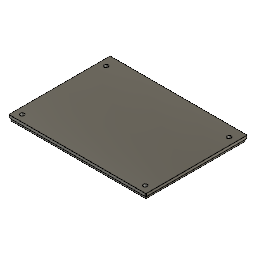
Final Board and Enclosure v2 (Autodesk Fusion 360 archive; units mm, degrees)
design "Lid"
Autodesk Fusion 360 part; units mm, degrees
sketch "Sketch 2" plane through (0, 0, 0) normal (0, 0, 1) x (1, 0, 0)
  circle A0 centre (5, 80) radius 1.75
  line L0 (-0.1, -0.1) -> (120.73, -0.1)
  arc A1 (-0.6, -1.1) -> (-1.1, -0.6) centre (-0.6, -0.6) cw
  line L1 (-1.1, -0.6) -> (-1.1, 89.17)
  arc A2 (-1.1, 89.17) -> (-0.6, 89.67) centre (-0.6, 89.17) cw
  line L2 (121.73, 89.17) -> (121.73, -0.6)
  circle A3 centre (115, 80) radius 1.75
  line L3 (120.73, -0.1) -> (120.73, 88.67)
  line L4 (120.73, 88.67) -> (-0.1, 88.67)
  circle A4 centre (115, 5) radius 1.75
  circle A5 centre (5, 5) radius 1.75
  line L5 (121.23, -1.1) -> (-0.6, -1.1)
  arc A6 (121.23, 89.67) -> (121.73, 89.17) centre (121.23, 89.17) cw
  line L6 (-0.1, 88.67) -> (-0.1, -0.1)
  arc A7 (121.73, -0.6) -> (121.23, -1.1) centre (121.23, -0.6) cw
  line L7 (-0.6, 89.67) -> (121.23, 89.67)
  line L8 (-0.1, 88.67) -> (120.73, 88.67)
  line L9 (120.73, 88.67) -> (120.73, -0.1)
  line L10 (120.73, -0.1) -> (-0.1, -0.1)
  line L11 (-0.1, -0.1) -> (-0.1, 88.67)
  dimension "d1" = 1
extrude "Extrude1" add sketch "Sketch 2" along normal blind 2.5 contours L0 L3 L4 L6 L8 L9 L10 L11 | A1 L1 A2 L2 L5 A6 A7 L7
extrude "Extrude2" add sketch "Sketch 2" against normal blind 2.5 contours L0 L3 L4 L6 L8 L9 L10 L11

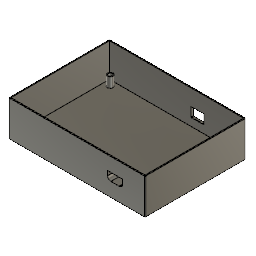
design "Enclosure PCB"
Autodesk Fusion 360 part; units mm, degrees
sketch "Sketch 1" plane through (0, 0, 0) normal (0, 0, 1) x (1, 0, 0)
  line L0 (-120.63, -88.57) -> (-120.63, 0)
  circle A0 centre (-115, -5) radius 1.75
  line L1 (0, 0) -> (0, -88.57)
  circle A1 centre (-115, -80) radius 1.75
  line L2 (-120.63, 0) -> (0, 0)
  circle A2 centre (-5, -80) radius 1.75
  line L3 (0, -88.57) -> (-120.63, -88.57)
  circle A3 centre (-5, -5) radius 1.75
  line L4 (0.1, -88.67) -> (-120.73, -88.67)
  line L5 (-120.73, -88.67) -> (-120.73, 0.1)
  line L6 (-120.73, 0.1) -> (0.1, 0.1)
  line L7 (0.1, 0.1) -> (0.1, -88.67)
  line L8 (1.1, -89.67) -> (-121.73, -89.67)
  line L9 (-121.73, -89.67) -> (-121.73, 1.1)
  line L10 (-121.73, 1.1) -> (1.1, 1.1)
  line L11 (1.1, 1.1) -> (1.1, -89.67)
  circle A4 centre (-115, -5) radius 2.5
  circle A5 centre (-115, -80) radius 2.5
  circle A6 centre (-5, -80) radius 2.5
  circle A7 centre (-5, -5) radius 2.5
  dimension "d1" = -0.1
  dimension "d2" = -1.1
  dimension "d7" = 5
  dimension "d8" = 5
  dimension "d9" = 5
  dimension "d10" = 5
  constraint concentric A0 A4
  constraint concentric A1 A5
  constraint concentric A2 A6
  constraint concentric A3 A7
  measures "d7" diameter of A4
  measures "d8" diameter of A5
  measures "d9" diameter of A6
  measures "d10" diameter of A7
extrude "Extrude1" add sketch "Sketch 1" against normal blind 2 contours L0 L1 L2 L3 | A0 | A1 | A2 | A3 | L8 L9 L10 L11 | A4 | A5 | A6 | A7 makes body 1 at (-40.21, -29.5233, 0) makes body 2 at (-40.1767, 0.7667, 0)
extrude "Extrude2" add sketch "Sketch 1" along normal blind 35 contours L8 L9 L10 L11 bodies 2
extrude "Extrude4" add sketch "Sketch 1" along normal blind 4 contours A4 | A5 | A6 | A7 bodies 1
extrude "Extrude5" add 4 faces at (-2.7658, -5.2111, 4) (-113.9872, -7.0026, 4) (-117.1045, -80.7791, 4) (-2.7593, -80.1242, 4) along direction (0, 0, 1) blind 3 on bodies 1 bodies 1
extrude "Extrude6" add 4 faces at (-113.9872, -7.0026, 7) (-2.7658, -5.2111, 7) (-117.1045, -80.7791, 7) (-2.7593, -80.1242, 7) along direction (0, 0, 1) blind 2 on bodies 1 bodies 1
extrude "Extrude7" cut 1 faces at (-40.1767, 0.7667, 35) along direction (0, 0, -1) blind 10 on bodies 2 bodies 2
extrude "Extrude8" add 1 faces at (-40.1767, 0.7667, 25) along direction (0, 0, 1) blind 5 on bodies 2 bodies 2
sketch "Sketch3" plane through (0, -89.67, 0) normal (0, -1, 0) x (1, 0, 0)
  line L0 (-121.73, 30) -> (-121.73, -2)
  line L1 (-121.73, -2) -> (1.1, -2)
  line L2 (1.1, -2) -> (1.1, 30)
  line L3 (1.1, 30) -> (-121.73, 30)
  line L4 (1.1, 5.8274) -> (-16.9, 5.8274) construction
  line L5 (-17.1151, -2) -> (-17.1151, 6) construction
  line L6 (-17.1151, 6) -> (-31.8464, 6)
  line L7 (-31.8464, 6) -> (-31.8464, 13)
  line L8 (-31.8464, 13) -> (-17.1151, 13)
  line L9 (-17.1151, 13) -> (-17.1151, 6)
  dimension "d23" = 18
  dimension "d24" = 8
  dimension "d25" = 7
  constraint coincident L2 L4.start
  constraint perpendicular L2 L4
  constraint coincident L1 L5.start
  constraint perpendicular L4 L5
  constraint horizontal L6
  constraint vertical L7
  constraint horizontal L8
  constraint vertical L9
  measures "d23" distance of L4.start L4.end
  measures "d24" distance of L5.start L5.end
  measures "d25" distance of L5.end L8.end
extrude "Extrude9" cut sketch "Sketch3" along normal blind 5.784 from surface at -1 contours L6 L7 L8 L9 bodies 2
extrude "Extrude10" add 1 faces at (-22.0255, -89.0033, 6) along direction (0, 0, 1) blind 2.752 on bodies 2 bodies 2
extrude "Extrude11" cut 1 faces at (-26.936, -89.0033, 13) along direction (0, 0, 1) blind 2.948 on bodies 2 bodies 2
extrude "Extrude12" cut 1 faces at (-26.936, -89.0033, 15.948) along direction (0, 0, 1) blind 1.69 on bodies 2 bodies 2
extrude "Extrude13" add 1 faces at (-22.0255, -89.0033, 8.752) along direction (0, 0, 1) blind 1.895 on bodies 2 bodies 2
extrude "Extrude14" add 1 faces at (-17.1151, -89.3367, 15.3077) along direction (-1, 0, 0) blind 2.086 on bodies 2 bodies 2
extrude "Extrude15" cut 1 faces at (-31.8464, -89.0033, 12.9773) along direction (-1, 0, 0) blind 0.829 on bodies 2 bodies 2
sketch "Sketch4" plane through (0, -88.67, 0) normal (0, 1, 0) x (-1, 0, 0)
  line L0 (32.6754, 10.647) -> (19.2011, 10.647)
  line L1 (19.2011, 10.647) -> (19.2011, 17.638)
  line L2 (19.2011, 17.638) -> (32.6754, 17.638)
  line L3 (32.6754, 17.638) -> (32.6754, 10.647)
  line L4 (-0.1, 30) -> (-0.1, -2)
  line L5 (-0.1, -2) -> (120.73, -2)
  line L6 (120.73, -2) -> (120.73, 30)
  line L7 (120.73, 30) -> (-0.1, 30)
  line L8 (18.4293, 18.3854) -> (33.6158, 18.3854)
  line L9 (33.6158, 18.3854) -> (33.6158, 9.7391)
  line L10 (33.6158, 9.7391) -> (18.4293, 9.7391)
  line L11 (18.4293, 9.7391) -> (18.4293, 18.3854)
  constraint horizontal L8
  constraint vertical L9
  constraint horizontal L10
  constraint vertical L11
extrude "Extrude16" add sketch "Sketch4" along normal blind 12.179 contours L8 L9 L10 L11 bodies 2
extrude "Extrude17" cut 1 faces at (-33.3023, -76.491, 12.9239) along direction (0, -1, 0) blind 6.186 on bodies 2 bodies 2
fillet "Fillet1" radius 0.5 1 edges at (1.1, 1.1, 14) on bodies 2
fillet "Fillet2" radius 0.5 1 edges at (1.1, -89.67, 14) on bodies 2
fillet "Fillet3" radius 0.5 1 edges at (-121.73, 1.1, 14) on bodies 2
fillet "Fillet4" radius 0.5 1 edges at (-121.73, -89.67, 14) on bodies 2
fillet "Fillet5" radius 3 1 edges at (-19.2011, -86.1735, 10.647) on bodies 2
fillet "Fillet6" radius 3 1 edges at (-32.6754, -86.1735, 10.647) on bodies 2
sketch "Sketch5" plane through (0, -82.677, 0) normal (0, 1, 0) x (-1, 0, 0)
  line L0 (19.2011, 17.638) -> (32.6754, 17.638)
  line L1 (32.6754, 17.638) -> (32.6754, 13.647)
  arc A0 (29.6754, 10.647) -> (32.6754, 13.647) centre (29.6754, 13.647) ccw
  line L2 (29.6754, 10.647) -> (22.2011, 10.647)
  arc A1 (19.2011, 13.647) -> (22.2011, 10.647) centre (22.2011, 13.647) ccw
  line L3 (19.2011, 13.647) -> (19.2011, 17.638)
  line L4 (18.4293, 9.7391) -> (33.6158, 9.7391)
  line L5 (33.6158, 9.7391) -> (33.6158, 18.3854)
  line L6 (33.6158, 18.3854) -> (18.4293, 18.3854)
  line L7 (18.4293, 18.3854) -> (18.4293, 9.7391)
  line L8 (19.2011, 17.638) -> (32.6754, 17.638)
  line L9 (32.6754, 17.638) -> (32.6754, 16.201)
  line L10 (32.6754, 16.201) -> (19.2011, 16.201)
  line L11 (19.2011, 16.201) -> (19.2011, 17.638)
  constraint horizontal L8
  constraint vertical L9
  constraint horizontal L10
  constraint vertical L11
  constraint coincident L1 L9.end
  constraint coincident L0.start L3.end
extrude "Extrude18" add sketch "Sketch5" along normal blind 2.383 separate body contours L0 L1 L3 L8 L9 L10 L11 makes body 3
sketch "Sketch6" plane through (0, -82.677, 0) normal (0, 1, 0) x (-1, 0, 0)
  line L0 (19.2011, 17.638) -> (32.6754, 17.638)
  line L1 (32.6754, 17.638) -> (32.6754, 13.647)
  arc A0 (29.6754, 10.647) -> (32.6754, 13.647) centre (29.6754, 13.647) ccw
  line L2 (29.6754, 10.647) -> (22.2011, 10.647)
  arc A1 (19.2011, 13.647) -> (22.2011, 10.647) centre (22.2011, 13.647) ccw
  line L3 (19.2011, 13.647) -> (19.2011, 17.638)
  line L4 (18.4293, 9.7391) -> (33.6158, 9.7391)
  line L5 (33.6158, 9.7391) -> (33.6158, 18.3854)
  line L6 (33.6158, 18.3854) -> (18.4293, 18.3854)
  line L7 (18.4293, 18.3854) -> (18.4293, 9.7391)
sketch "Sketch7" plane through (0, -82.677, 0) normal (0, 1, 0) x (-1, 0, 0)
sketch "Sketch8" plane through (0, -82.677, 0) normal (0, 1, 0) x (-1, 0, 0)
sketch "Sketch9" plane through (0, -82.677, 0) normal (0, 1, 0) x (-1, 0, 0)
sketch "Sketch10" plane through (0, -88.67, 0) normal (0, 1, 0) x (-1, 0, 0)
sketch "Sketch11" plane through (0, 1.1, 0) normal (0, 1, 0) x (-1, 0, 0)
  line L0 (121.23, -2) -> (121.23, 30)
  line L1 (121.23, 30) -> (-0.6, 30)
  line L2 (-0.6, 30) -> (-0.6, -2)
  line L3 (-0.6, -2) -> (121.23, -2)
  line L4 (19.1502, 15.374) -> (32.0205, 15.374)
  line L5 (32.0205, 15.374) -> (32.0205, 4.3423)
  line L6 (32.0205, 4.3423) -> (19.1502, 4.3423)
  line L7 (19.1502, 4.3423) -> (19.1502, 15.374)
  constraint horizontal L4
  constraint vertical L5
  constraint horizontal L6
  constraint vertical L7
extrude "Extrude19" cut sketch "Sketch11" along normal blind 7.369 from surface at -1 contours L4 L5 L6 L7 bodies 2
extrude "Extrude20" cut 1 faces at (-32.0205, 0.4333, 11.6967) along direction (-1, 0, 0) blind 22.557 on bodies 2 bodies 2
extrude "Extrude21" add 1 faces at (-19.1502, 0.4333, 8.0195) along direction (-1, 0, 0) blind 20.425 on bodies 2 bodies 2
extrude "Extrude22" cut 1 faces at (-39.5752, 0.4333, 8.0195) along direction (1, 0, 0) blind 4.126 on bodies 2 bodies 2
extrude "Extrude23" add 1 faces at (-54.5775, 0.4333, 11.6967) along direction (1, 0, 0) blind 5.127 on bodies 2 bodies 2
extrude "Extrude24" add 1 faces at (-44.7834, 0.4333, 4.3423) along direction (0, 0, 1) blind 0.064 on bodies 2 bodies 2
extrude "Extrude25" add 1 faces at (-49.4505, 0.4333, 11.7181) along direction (1, 0, 0) blind 2.072 on bodies 2 bodies 2
extrude "Extrude26" add 1 faces at (-35.4492, 0.7667, 8.0622) along direction (-1, 0, 0) blind 0.46 on bodies 2 bodies 2
extrude "Extrude27" add 1 faces at (-43.5554, 0.7667, 4.4063) along direction (0, 0, 1) blind 1.078 on bodies 2 bodies 2
extrude "Extrude28" add 1 faces at (-43.5554, 0.7667, 5.4843) along direction (0, 0, 1) blind 1.458 on bodies 2 bodies 2
sketch "Sketch12" plane through (0, 1.1, 0) normal (0, 1, 0) x (-1, 0, 0)
  line L0 (35.9092, 15.374) -> (47.3785, 15.374)
  line L1 (47.3785, 15.374) -> (47.3785, 6.9423)
  line L2 (47.3785, 6.9423) -> (35.9092, 6.9423)
  line L3 (35.9092, 6.9423) -> (35.9092, 15.374)
  line L4 (121.23, -2) -> (121.23, 30)
  line L5 (121.23, 30) -> (-0.6, 30)
  line L6 (-0.6, 30) -> (-0.6, -2)
  line L7 (-0.6, -2) -> (121.23, -2)
  line L8 (35.2835, 16.0008) -> (47.986, 16.0008)
  line L9 (47.986, 16.0008) -> (47.986, 6.3931)
  line L10 (47.986, 6.3931) -> (35.2835, 6.3931)
  line L11 (35.2835, 6.3931) -> (35.2835, 16.0008)
  dimension "d74" = 12.7025
  constraint horizontal L8
  constraint vertical L9
  constraint horizontal L10
  constraint vertical L11
  measures "d74" distance of L8.start L8.end
extrude "Extrude29" add sketch "Sketch12" along normal blind 1.287 contours L8 L9 L10 L11 bodies 2
extrude "Extrude3" [suppressed]
